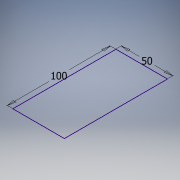
# Autodesk Inventor part: Mid
Saved by Autodesk Inventor 2019 (Build 230136000, 136)
## iProperties
Created: 2019-11-04
Part Number: Mid
Material: Generic
Document SubType Name: Modeling
Designer: Mark
Density: 1 g/cm^3
Appearance: Default
Author: Mark
Autodesk Inventor part; units mm, degrees
ref_plane "YZ Plane" through (0, 0, 0) normal (1, 0, 0) x (0, 1, 0)
ref_plane "XZ Plane" through (0, 0, 0) normal (0, 1, 0) x (-1, 0, 0)
ref_plane "XY Plane" through (0, 0, 0) normal (0, 0, 1) x (1, 0, 0)
sketch "Sketch1" plane through (0, 0, 0) normal (0, 1, 0) x (-1, 0, 0)
  line L0 (50, -10) -> (-50, -10)
  line L1 (-50, -10) -> (-50, 10)
  line L2 (-50, 10) -> (50, 10)
  line L3 (50, 10) -> (50, -10)
  line L4 (50, -10) -> (-50, 10) construction
  line L5 (-50, -10) -> (50, 10) construction
  line L6 (48, -8) -> (-48, -8)
  line L7 (-48, -8) -> (-48, 8)
  line L8 (-48, 8) -> (48, 8)
  line L9 (48, 8) -> (48, -8)
  line L10 (48, -8) -> (-48, 8) construction
  line L11 (-48, -8) -> (48, 8) construction
  point P0 (0, 0)
  dimension "d2" = 100
  dimension "d3" = 20
  dimension "d4" = 96
  dimension "d5" = 16
  constraints: 24 end point, 4 midpoint, 4 parallel, 2 horizontal, 2 perpendicular
  measures "d2" distance of L1.end L2.end
  measures "d3" distance of L0.end L1.end
  measures "d4" distance of L7.end L8.end
  measures "d5" distance of L6.end L7.end
extrude "Extrusion1" add sketch "Sketch1" along normal blind 448
body "Solid1"
